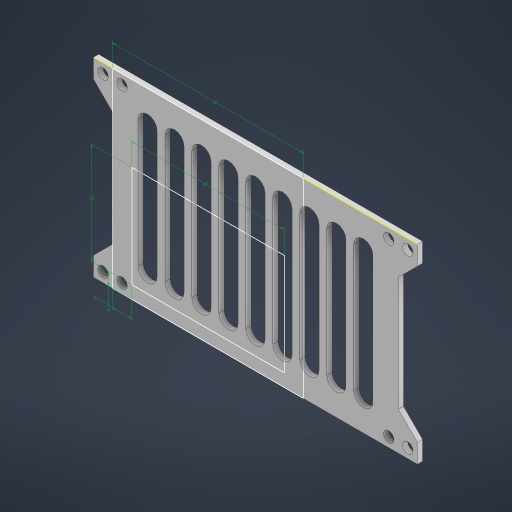
# Autodesk Inventor part: IntakeFilterTop
Saved by Autodesk Inventor 2024.2 (Build 282272000, 272)
## iProperties
Created: 2024-06-05
Part Number: IntakeFilterTop
Material: Generic
Document SubType Name: Modeling
Designer: simon
Density: 1 g/cm^3
Appearance: Default
Author: simon
Autodesk Inventor part; units mm, degrees
ref_plane "YZ Plane" through (0, 0, 0) normal (1, 0, 0) x (0, 1, 0)
ref_plane "XZ Plane" through (0, 0, 0) normal (0, 1, 0) x (-1, 0, 0)
ref_plane "XY Plane" through (0, 0, 0) normal (0, 0, 1) x (1, 0, 0)
sketch "Sketch1" plane through (0, 0, 0) normal (0, 0, 1) x (1, 0, 0)
  line L0 (0, 0) -> (90, 0)
  line L1 (90, 0) -> (90, 60)
  line L2 (90, 60) -> (0, 60)
  line L3 (0, 60) -> (0, 0)
  line L4 (-10, 30) -> (100, 30)
  line L5 (8, 10) -> (8, 50)
  line L6 (14, 10) -> (14, 50)
  arc A0 (14, 50) -> (8, 50) centre (11, 50) ccw
  arc A1 (8, 10) -> (14, 10) centre (11, 10) ccw
  arc A2 (22.5, 50) -> (16.5, 50) centre (19.5, 50) ccw
  line L7 (16.5, 10) -> (16.5, 50)
  line L8 (22.5, 10) -> (22.5, 50)
  arc A3 (16.5, 10) -> (22.5, 10) centre (19.5, 10) ccw
  arc A4 (31, 50) -> (25, 50) centre (28, 50) ccw
  line L9 (25, 10) -> (25, 50)
  line L10 (31, 10) -> (31, 50)
  arc A5 (25, 10) -> (31, 10) centre (28, 10) ccw
  arc A6 (39.5, 50) -> (33.5, 50) centre (36.5, 50) ccw
  line L11 (33.5, 10) -> (33.5, 50)
  line L12 (39.5, 10) -> (39.5, 50)
  arc A7 (33.5, 10) -> (39.5, 10) centre (36.5, 10) ccw
  arc A8 (48, 50) -> (42, 50) centre (45, 50) ccw
  line L13 (42, 10) -> (42, 50)
  line L14 (48, 10) -> (48, 50)
  arc A9 (42, 10) -> (48, 10) centre (45, 10) ccw
  arc A10 (56.5, 50) -> (50.5, 50) centre (53.5, 50) ccw
  line L15 (50.5, 10) -> (50.5, 50)
  line L16 (56.5, 10) -> (56.5, 50)
  arc A11 (50.5, 10) -> (56.5, 10) centre (53.5, 10) ccw
  line L17 (0, 60) -> (-6, 60)
  line L18 (-6, 60) -> (-6, 54)
  line L19 (-6, 54) -> (0, 48)
  line L20 (0, 0) -> (-6, 0)
  line L21 (-6, 0) -> (-6, 6)
  line L22 (-6, 6) -> (0, 12)
  line L23 (90, 60) -> (96, 60)
  line L24 (96, 60) -> (96, 54)
  line L25 (96, 54) -> (90, 48)
  line L26 (90, 0) -> (96, 0)
  line L27 (96, 0) -> (96, 6)
  line L28 (96, 6) -> (90, 12)
  circle A12 centre (3, 57) radius 1.65
  circle A13 centre (-3, 57) radius 1.65
  line L29 (45, 72.0135) -> (45, -11.3556)
  circle A14 centre (93, 57) radius 1.65
  circle A15 centre (-3, 3) radius 1.65
  circle A16 centre (93, 3) radius 1.65
  circle A17 centre (87, 57) radius 1.65
  circle A18 centre (3, 3) radius 1.65
  circle A19 centre (87, 3) radius 1.65
  arc A20 (65, 50) -> (59, 50) centre (62, 50) ccw
  line L30 (59, 10) -> (59, 50)
  line L31 (65, 10) -> (65, 50)
  arc A21 (59, 10) -> (65, 10) centre (62, 10) ccw
  arc A22 (73.5, 50) -> (67.5, 50) centre (70.5, 50) ccw
  line L32 (67.5, 10) -> (67.5, 50)
  line L33 (73.5, 10) -> (73.5, 50)
  arc A23 (67.5, 10) -> (73.5, 10) centre (70.5, 10) ccw
  arc A24 (82, 50) -> (76, 50) centre (79, 50) ccw
  line L34 (76, 10) -> (76, 50)
  line L35 (82, 10) -> (82, 50)
  arc A25 (76, 10) -> (82, 10) centre (79, 10) ccw
  dimension "d0" = 90
  dimension "d1" = 60
  dimension "d2" = 110
  dimension "d3" = 60
  dimension "d4" = 10
  dimension "d5" = 8
  dimension "d6" = 6
  dimension "d7" = 40
  dimension "d8" = 40
  dimension "d9" = 10
  dimension "d10" = 10
  dimension "d13" = 8.5
  dimension "d18" = 6
  dimension "d19" = 6
  dimension "d20" = 6
  dimension "d21" = 6
  dimension "d22" = 6
  dimension "d23" = 6
  dimension "d24" = 6
  dimension "d25" = 6
  dimension "d26" = 6
  dimension "d27" = 6
  dimension "d28" = 6
  dimension "d29" = 6
  dimension "d30" = 3.3
  dimension "d31" = 3.3
  dimension "d32" = 3
  dimension "d33" = 3
  dimension "d34" = 90
  dimension "d37" = 96
  dimension "d40" = 54
  dimension "d43" = 3
  dimension "d44" = 3
  dimension "d47" = 84
  dimension "d50" = 54
  constraints: 72 end point, 36 point on circle, 26 centre point, 9 horizontal, 5 perpendicular, 5 vertical, 4 point on line, 2 parallel, 2 tangent, 92 other
  measures "d0" distance of L2.end L1.end
  measures "d1" distance of L1.end L0.end
  measures "d2" distance of L4.start L4.end
  measures "d3" diameter of L0.start L4
  measures "d4" distance from line of L3 L4.start
  measures "d5" distance between parallel lines of L3 L5
  measures "d6" distance between parallel lines of L6 L5
  measures "d7" distance of L5.start L5.end
  measures "d8" distance of L6.start L6.end
  measures "d9" distance from line of L0 L5.start
  measures "d10" distance from line of L0 L6.start
  measures "d13" distance of A0.centre A2.centre
  measures "d18" distance of L17.end L18.end
  measures "d19" distance of L2.end L17.end
  measures "d20" horizontal distance of L19.end L18.end
  measures "d21" distance of L20.end L21.end
  measures "d22" distance of L0.start L20.end
  measures "d23" horizontal distance of L22.end L21.end
  measures "d24" distance of L1.end L23.end
  measures "d25" distance of L23.end L24.end
  measures "d26" horizontal distance of L25.end L24.end
  measures "d27" distance of L26.end L27.end
  measures "d28" distance of L0.end L26.end
  measures "d29" horizontal distance of L28.end L27.end
  measures "d30" diameter of A12
  measures "d31" diameter of A13
  measures "d32" distance from line of L17 A13.centre
  measures "d33" distance from line of L18 A13.centre
  measures "d34" diameter of L3 L29
  measures "d37" distance of A13.centre A14.centre
  measures "d40" distance of A13.centre A15.centre
  measures "d43" distance from line of L2 A12.centre
  measures "d44" distance from line of L3 A12.centre
  measures "d47" distance of A12.centre A17.centre
  measures "d50" distance of A12.centre A18.centre
extrude "Extrusion1" add sketch "Sketch1" along normal blind 1.6 contours L3 L4 L5 A1 L6 L7 A3 L8 L9 A5 L10 L11 A7 L12 L13 A9 L29 L0 | L20 L21 L22 L3 | L29 A9 L14 L4 L15 A11 L16 L30 A21 L31 L32 A23 L33 L34 A25 L35 L1 L0 | L1 L28 L27 L26 | L3 L2 L29 A8 L13 L4 L12 A6 L11 L10 A4 L9 L8 A2 L7 L6 A0 L5 | L19 L18 L17 L3 | L4 L35 A24 L34 L33 A22 L32 L31 A20 L30 L16 A10 L15 L14 A8 L29 L2 L1 | L1 L23 L24 L25
sketch "Sketch2" plane through (0, 0, 1.6) normal (0, 0, 1) x (1, 0, 0)
  line L0 (96, 60) -> (-6, 60) projected
  line L1 (0, 0) -> (60, 0)
  line L2 (60, 0) -> (60, 60)
  line L3 (60, 60) -> (0, 60)
  line L4 (0, 60) -> (0, 0)
  line L5 (6, 4) -> (54, 4)
  line L6 (54, 4) -> (54, 36)
  line L7 (54, 36) -> (6, 36)
  line L8 (6, 36) -> (6, 4)
  dimension "d55" = 60
  dimension "d56" = 48
  dimension "d57" = 32
  dimension "d58" = 4
  dimension "d59" = 6
  constraints: 16 end point, 4 parallel, 2 horizontal, 2 perpendicular, 1 point on line
  measures "d55" distance between parallel lines of L2 L4
  measures "d56" distance of L6.end L7.end
  measures "d57" distance of L7.end L5.start
  measures "d58" distance between parallel lines of L5 L1
  measures "d59" distance between parallel lines of L4 L8
body "Solid1"
